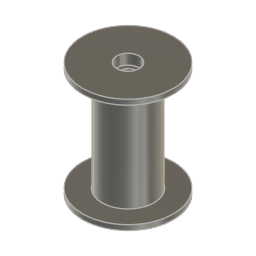
BushingPulley60AIM_HGR (Autodesk Fusion 360 design; units mm, degrees)
Autodesk Fusion 360 part; units mm, degrees
note: some values were not read from the file. Set by a fixed rule: which sketch regions a step uses.
sketch "Sketch1" plane through (0, 0, 0) normal (0, 0, 1) x (1, 0, 0)
  circle A0 centre (0, 0) radius 10.05
  line L0 (2.35, -4.2) -> (2.35, -9.4)
  line L1 (-2.35, -4.2) -> (2.35, -4.2)
  line L2 (-2.35, -4.2) -> (2.35, -9.4) construction
  line L3 (2.35, -9.4) -> (-2.35, -9.4)
  line L4 (2.35, -4.2) -> (-2.35, -9.4) construction
  line L5 (-2.35, -9.4) -> (-2.35, -4.2)
  circle A1 centre (0, 0) radius 7.1
  circle A2 centre (0, 0) radius 17.5
  line L6 (0, 0) -> (0, -12)
  point P0 (0, -6.8)
  dimension "d1" = 20.1
  dimension "d2" = 4.7
  dimension "d3" = 5.2
  dimension "d4" = 14.2
  dimension "d5" = 2.9
  dimension "d10" = 35
  constraint coincident A0.centre A1.centre
  constraint horizontal L1
  constraint perpendicular L0 L1
  constraint parallel L1 L3
  constraint parallel L0 L5
  constraint coincident P0 L2
  constraint coincident P0 L4
  constraint perpendicular L3 L6
  constraint coincident P0 L6
  measures "d1" diameter of A0
  measures "d2" distance of L3.end L0.end
  measures "d3" distance of L0.end L0.start
  measures "d4" diameter of A1
  measures "d5" distance of L1 A1
  measures "d10" diameter of A2
extrude "Extrude1" add sketch "Sketch1" along normal blind 42 contours A0 | L0 L1 A1 L6 | L0 L3 A1 L6 | L1 L5 A1 L6 | L3 L5 A1 L6 makes body 1
extrude "Extrude2" add sketch "Sketch1" along normal blind 2 contours A2 bodies 1
extrude "Extrude3" add sketch "Sketch1" along normal blind 2 from surface at 42 separate body contours A0 | L0 L1 A1 L6 | L0 L3 A1 L6 | L1 L5 A1 L6 | L3 L5 A1 L6 | A2 makes body 2
extrude "Extrude4" add sketch "Sketch1" against normal blind 20 from surface at 44 separate body contours L0 L1 L5 A1 | L0 L1 A1 L6 | L1 L5 A1 L6 makes body 3
combine "Combine1" operation add target body 2 tool bodies 3
move_face "OffsetFaces1" [suppressed]
sketch "Sketch2" plane through (0, 0, 44) normal (0, 0, 1) x (-1, 0, 0)
  circle A0 centre (0, 0) radius 17.5
  circle A1 centre (0, 0) radius 3
  constraint concentric A0 A1
extrude "Extrude5" cut sketch "Sketch1" against normal blind 18 from surface at 42 contours L0 L1 A1 L6 | L1 L5 A1 L6 bodies 1
hole "Hole1" at (0, 0, 44) direction (0, 0, -1) diameter 5.4 depth 65 tip angle 118 counterbore diameter 8.6 counterbore depth 4 bodies 2
extrude "Extrude6" cut sketch "Sketch1" along normal blind 7 contours L0 L1 A1 L6 | L1 L5 A1 L6 bodies 1
